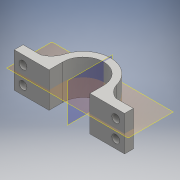
# Autodesk Inventor part: Motor Mount
Saved by Autodesk Inventor 2016 (Build 200138000, 138)
## iProperties
Created: 2016-04-05
Part Number: Motor Mount
Material: Generic
Document SubType Name: Modeling
Designer: Kenneth Daniel
Density: 1 g/cm^3
Appearance: Default
Author: Kenneth Daniel
Autodesk Inventor part; units mm, degrees
ref_plane "YZ Plane" through (0, 0, 0) normal (1, 0, 0) x (0, 1, 0)
ref_plane "XZ Plane" through (0, 0, 0) normal (0, 1, 0) x (-1, 0, 0)
ref_plane "XY Plane" through (0, 0, 0) normal (0, 0, 1) x (1, 0, 0)
sketch "Sketch1" plane through (0, 0, 0) normal (0, 0, 1) x (1, 0, 0)
  line L0 (88, 5) -> (88, 7)
  line L1 (0, 7) -> (0, 5)
  line L2 (0, 0) -> (0, 32) construction
  line L3 (0, 32) -> (28, 32) construction
  line L4 (28, 32) -> (60, 32) construction
  line L5 (60, 32) -> (88, 32) construction
  line L6 (88, 32) -> (88, 0) construction
  line L7 (60, 63.7192) -> (60, -36.6397) construction
  line L8 (28, 67.21) -> (28, -43.6212) construction
  line L9 (44, 32) -> (44, 16) construction
  line L10 (27.7, 5) -> (27.7, 16)
  arc A0 (60.3, 16) -> (27.7, 16) centre (44, 16) ccw
  line L11 (60.3, 16) -> (60.3, 5)
  arc A1 (65.223, 20.9825) -> (22.777, 20.9825) centre (44, 16) ccw
  line L12 (22.2, 7) -> (13.2, 7)
  line L13 (22.2, 0) -> (22.2, 5)
  line L14 (22.2, 5) -> (0, 5)
  line L15 (0, 5) -> (0, 12)
  line L16 (88, 12) -> (88, 5)
  line L17 (22.2, 7) -> (13.2, 7)
  arc A2 (14, 12) -> (22.777, 20.9825) centre (8.2155, 26.4316) ccw
  arc A3 (65.223, 20.9825) -> (74, 12) centre (79.7845, 26.4316) ccw
  line L18 (60.3, 7) -> (60, 7)
  line L19 (28, 7) -> (27.7, 7)
  line L20 (22.2, 5) -> (28, 5)
  line L21 (60, 5) -> (88, 5)
  line L22 (27.7, 0) -> (28, 0)
  line L23 (60, 0) -> (60.3, 0)
  line L24 (0, 12) -> (14, 12)
  line L25 (27.7, 12) -> (28, 12)
  line L26 (22.2, 0) -> (22.2, 7)
  line L27 (60, 12) -> (60.3, 12)
  line L28 (74, 12) -> (88, 12)
  dimension "d0" = 88
  dimension "d1" = 7
  dimension "d2" = 32
  dimension "d3" = 28
  dimension "d4" = 32
  dimension "d5" = 28
  dimension "d6" = 16
  dimension "d8" = 5.5
  dimension "d9" = 9
  dimension "d10" = 5
  dimension "d11" = 7
  dimension "d12" = 9
  constraints: 58 end point, 25 point on line, 12 perpendicular, 8 point on circle, 4 centre point, 4 vertical, 3 horizontal, 3 symmetric about line, 1 coincident, 1 midpoint, 1 other
  measures "d0" distance of L2.start L6.end
  measures "d1" distance of L6.end L0.end
  measures "d2" distance of L2.start L2.end
  measures "d3" distance of L2.end L3.end
  measures "d4" distance of L3.end L4.end
  measures "d5" distance of L4.end L5.end
  measures "d6" distance of L9.start L9.end
  measures "d8" radial gap between concentric circles of A0 A1
  measures "d9" distance of L12.start L12.end
  measures "d10" distance of L13.start L13.end
  measures "d11" distance of L1.end L15.end
  measures "d12" distance of L12.start L12.end
extrude "Extrusion1" add sketch "Sketch1" along normal blind 28
sketch "Sketch2" plane through (0, 12, 0) normal (0, 1, 0) x (1, 0, 0)
  line L0 (14, 0) -> (0, 0) projected
  line L1 (14, 0) -> (14, -28) projected
  line L2 (0, 0) -> (14, -28) construction
  line L3 (14, 0) -> (0, -28) construction
  line L4 (7, 0) -> (7, -7) construction
  circle A0 centre (7, -7) radius 2.743
  dimension "d15" = 7
  dimension "d16" = 5.486
  constraints: 6 end point, 1 centre point, 1 coincident, 1 midpoint, 1 vertical
  measures "d15" distance of L4.start L4.end
  measures "d16" diameter of A0
extrude "Extrusion2" cut sketch "Sketch2" against normal blind 28
ref_plane "Work Plane1" through (0, 0, 14) normal (0, 0, 1) x (1, 0, 0)
ref_plane "Work Plane2" through (44, 5, 0) normal (-1, 0, 0) x (0, 0, 1)
mirror "Mirror1" about plane through (0, 0, 14) normal (0, 0, 1) of "Extrusion2"
mirror "Mirror2" about plane through (44, 5, 0) normal (-1, 0, 0) of "Extrusion2", "Mirror1"
sketch "Sketch3" plane through (0, 12, 0) normal (0, 1, 0) x (1, 0, 0)
  circle A0 centre (7, -21) radius 2.743 projected
  circle A1 centre (7, -7) radius 2.743 projected
  line L0 (14, 0) -> (0, 0) projected
  line L1 (0, 0) -> (0, -28) projected
  line L2 (14, -28) -> (0, -28) projected
  line L3 (14, 0) -> (14, -28) projected
  circle A2 centre (7, -7) radius 3.143
  circle A3 centre (7, -7) radius 2.743
  dimension "d19" = 0.4
  constraints: 2 centre point, 1 coincident, 1 concentric
  measures "d19" radial gap between concentric circles of A1 A2
extrude "Extrusion3" cut sketch "Sketch3" against normal blind 10 contours A2
mirror "Mirror3" about plane through (0, 0, 14) normal (0, 0, 1) of "Extrusion3"
mirror "Mirror4" about plane through (44, 5, 0) normal (-1, 0, 0) of "Extrusion3", "Mirror3"
body "Solid1"
